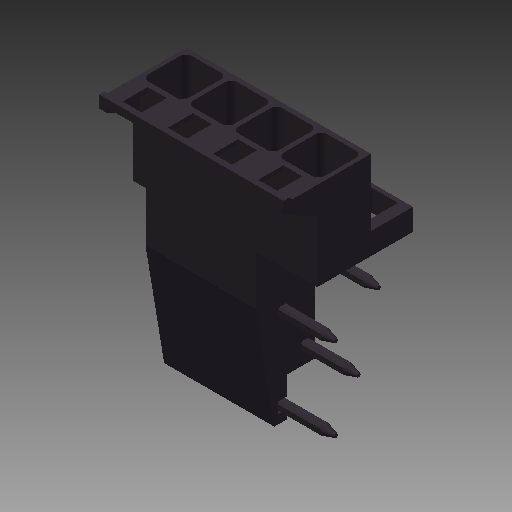
# Autodesk Inventor part: SHL-SMT5.00/04/GL 5.9BX 1069770000
Saved by Autodesk Inventor 2019.3 (Build 233278000, 278)
## iProperties
Category: PARTsolutions
Company: WEIDMUELLER
Created: 2018-11-15
Part Number: SHL-SMT5.00/04/GL 5.9BX 1069770000
Material: Generic
Catalog Web Link: www.cadenas.de
Description: SHL-SMT5.00/GL-Electronics housings
Vendor: WEIDMUELLER
Document SubType Name: Modeling
Designer: psadmin
Manufacturer: WEIDMUELLER
Mass: 1.86348 g
Surface Area: 26.7097 cm^2
Volume: 1.86348 cm^3
Density: 1 g/cm^3
Appearance: PSOLRGB-68-61-68
PSOL_IDENT_0: {$CADENAS_DATA\23d-libs\weidmueller\elektronikgehaeuse\einbaugehaeuse\ch20m\zubehoer\shl-smt500_gl.p
PSOL_IDENT_1: rj},216 {VTYP=3D},{NB=SHL-SMT5.00/04/GL 5.9BX 1069770000},{LINA=SHL-SMT5.00/04/GL 5.9BX 1069770000},
PSOL_IDENT_2: {NN=SHL-SMT5.00/GL},{DATE=31.03.2017 09:22:38},{GEOMDATE=25.06.2010 07:04:00},{VERSION=},{LINEID=50}
PSOL_IDENT_3: ,{WBVAR=},{WBNUMERIC=}  {NB=SHL-SMT5.00/04/GL 5.9BX 1069770000},{LINA=SHL-SMT5.00/04/GL 5.9BX 106977
PSOL_IDENT_4: 0000},{KT=DUMMY},{BEST=1069770000},{BZ=SHL-SMT5.00/04/GL 5.9BX},{R=5.00},{P=4},{L=5.90},{F=schwarz},
PSOL_IDENT_5: {FCODE=0.27,0.24,0.27,0.00}
NN: SHL-SMT5.00/GL
NT: Electronics housings
NB: SHL-SMT5.00/04/GL 5.9BX 1069770000
NBSYN: $BZ. $BEST.
LINA: SHL-SMT5.00/04/GL 5.9BX 1069770000
BEST: 1069770000
BZ: SHL-SMT5.00/04/GL 5.9BX
R: 5
P: 4
L: 5.9
F: black
SUPPLIER: WEIDMUELLER
ARTICLENO: SHL-SMT5.00/04/GL 5.9BX 1069770000
BOMINFO: SHL-SMT5.00/04/GL 5.9BX 1069770000
CREATOR: CADENAS GmbH
Title: SHL-SMT5.00/04/GL 5.9BX 1069770000
Author: Cadenas PARTsolutions
Comments: Electronics housings
Autodesk Inventor part; units mm, degrees
sketch "Sketch_2" plane through (-15.2, 0, 0) normal (1, 0, 0) x (0, 0, -1)
  line L0 (-14.35, 12.05) -> (-14.35, 10.7061)
  line L1 (-14.35, 10.7061) -> (-10.6, 8.67)
  line L2 (-10.6, 8.67) -> (-10.6, -3.6)
  line L3 (-10.6, -3.6) -> (-8.5417, -15.9)
  line L4 (-8.5417, -15.9) -> (-7.1, -15.9)
  line L5 (-7.1, -15.9) -> (-7.1, -11.6)
  line L6 (-7.1, -11.6) -> (-4.1, -11.6)
  line L7 (-4.1, -11.6) -> (-4.1, -4.05)
  line L8 (-4.1, -4.05) -> (-1.85, -4.05)
  line L9 (-1.85, -4.05) -> (-1.85, 1.9)
  line L10 (-1.85, 1.9) -> (0, 1.9)
  line L11 (0, 1.9) -> (0, 4.3)
  line L12 (0, 4.3) -> (-4.64, 4.3)
  line L13 (-4.64, 4.3) -> (-4.64, 11.7)
  line L14 (-4.64, 11.7) -> (-13.375, 11.7)
  line L15 (-13.375, 11.7) -> (-13.725, 12.05)
  line L16 (-13.725, 12.05) -> (-14.35, 12.05)
  constraints: 34 end point
extrude "Extrusion1" add sketch "Sketch_2" along normal blind 20.4
sketch "Sketch_4" plane through (0, 0, 0) normal (0, 0, 1) x (1, 0, 0)
  line L0 (-1.6, -16) -> (5.4, -16)
  line L1 (5.4, -16) -> (5.4, 1.9)
  line L2 (5.4, 1.9) -> (-1.6, 1.9)
  line L3 (-1.6, 1.9) -> (-1.6, -16)
  constraints: 8 end point
extrude "Extrusion2" cut sketch "Sketch_4" along normal blind 11
sketch "Sketch_15" plane through (0, 0, 0) normal (0, 0, 1) x (1, 0, 0)
  line L0 (-15.5, -5.1) -> (-6.5, -5.1)
  line L1 (-6.5, -5.1) -> (-6.5, 1.9)
  line L2 (-6.5, 1.9) -> (-15.5, 1.9)
  line L3 (-15.5, 1.9) -> (-15.5, -5.1)
  constraints: 8 end point
extrude "Extrusion3" cut sketch "Sketch_15" along normal blind 4.1
sketch "Sketch_13" plane through (0, 11.7, 0) normal (0, 1, 0) x (1, 0, 0)
  line L0 (0.25, -5.825) -> (0.25, -9.375)
  arc A0 (0.25, -9.375) -> (0.9, -10.025) centre (0.9, -9.375) ccw
  line L1 (0.9, -10.025) -> (4.1, -10.025)
  arc A1 (4.1, -10.025) -> (4.75, -9.375) centre (4.1, -9.375) ccw
  line L2 (4.75, -9.375) -> (4.75, -5.825)
  arc A2 (4.75, -5.825) -> (4.1, -5.175) centre (4.1, -5.825) ccw
  line L3 (4.1, -5.175) -> (0.9, -5.175)
  arc A3 (0.9, -5.175) -> (0.25, -5.825) centre (0.9, -5.825) ccw
  constraints: 8 end point, 8 point on circle, 4 centre point
extrude "Extrusion4" cut sketch "Sketch_13" against normal blind 8.7
pattern_linear "Rectangular Pattern1" count 4 spacing 5 along (-1, 0, 0) of "Extrusion4"
sketch "Sketch_21" plane through (0, 11.7, 0) normal (0, 1, 0) x (1, 0, 0)
  line L0 (1.45, -10.6) -> (1.45, -13.375)
  line L1 (1.45, -13.375) -> (3.55, -13.375)
  line L2 (3.55, -13.375) -> (3.55, -10.6)
  line L3 (3.55, -10.6) -> (1.45, -10.6)
  constraints: 8 end point
extrude "Extrusion5" cut sketch "Sketch_21" against normal blind 4
pattern_linear "Rectangular Pattern2" count 4 spacing 5 along (-1, 0, 0) of "Extrusion5"
sketch "Sketch_23" plane through (-14.4, 0, 0) normal (1, 0, 0) x (0, 0, -1)
  line L0 (-14.6, 8.2) -> (-10.6, 8.2)
  line L1 (-10.6, 8.2) -> (-10.6, 11.2)
  line L2 (-10.6, 11.2) -> (-14.6, 11.2)
  line L3 (-14.6, 11.2) -> (-14.6, 8.2)
  constraints: 8 end point
extrude "Extrusion6" cut sketch "Sketch_23" along normal blind 18.8
sketch "Sketch_28" plane through (0, 4.3, 0) normal (0, 1, 0) x (1, 0, 0)
  line L0 (1, -0.65) -> (1, -3.65)
  arc A0 (1, -3.65) -> (1.2, -3.85) centre (1.2, -3.65) ccw
  line L1 (1.2, -3.85) -> (3.8, -3.85)
  arc A1 (3.8, -3.85) -> (4, -3.65) centre (3.8, -3.65) ccw
  line L2 (4, -3.65) -> (4, -0.65)
  arc A2 (4, -0.65) -> (3.8, -0.45) centre (3.8, -0.65) ccw
  line L3 (3.8, -0.45) -> (1.2, -0.45)
  arc A3 (1.2, -0.45) -> (1, -0.65) centre (1.2, -0.65) ccw
  constraints: 8 end point, 8 point on circle, 4 centre point
extrude "Extrusion7" cut sketch "Sketch_28" against normal blind 2.4
sketch "Sketch_29" plane through (0, 4.3, 0) normal (0, 1, 0) x (1, 0, 0)
  line L0 (-14, -0.65) -> (-14, -3.65)
  arc A0 (-14, -3.65) -> (-13.8, -3.85) centre (-13.8, -3.65) ccw
  line L1 (-13.8, -3.85) -> (-11.2, -3.85)
  arc A1 (-11.2, -3.85) -> (-11, -3.65) centre (-11.2, -3.65) ccw
  line L2 (-11, -3.65) -> (-11, -0.65)
  arc A2 (-11, -0.65) -> (-11.2, -0.45) centre (-11.2, -0.65) ccw
  line L3 (-11.2, -0.45) -> (-13.8, -0.45)
  arc A3 (-13.8, -0.45) -> (-14, -0.65) centre (-13.8, -0.65) ccw
  constraints: 8 end point, 8 point on circle, 4 centre point
extrude "Extrusion8" cut sketch "Sketch_29" against normal blind 2.4
sketch "Sketch_10" plane through (0, 0, 7.1) normal (0, 0, 1) x (1, 0, 0)
  line L0 (-13.1, 1.9) -> (-13.1, -13.2)
  arc A0 (-13.1, -13.2) -> (-11.4, -14.9) centre (-11.4, -13.2) ccw
  line L1 (-11.4, -14.9) -> (-1.6, -14.9)
  line L2 (-1.6, -14.9) -> (-1.6, -13.7)
  line L3 (-1.6, -13.7) -> (-11.4, -13.7)
  arc A1 (-11.9, -13.2) -> (-11.4, -13.7) centre (-11.4, -13.2) ccw
  line L4 (-11.9, -13.2) -> (-11.9, 1.9)
  line L5 (-11.9, 1.9) -> (-13.1, 1.9)
  constraints: 12 end point, 4 point on circle, 2 centre point
extrude "Extrusion9" cut sketch "Sketch_10" along normal blind 1
sketch "Sketch_5" plane through (4.3, 0, 0) normal (1, 0, 0) x (0, 0, -1)
  line L0 (-8.1, -4.9) -> (-8.1, -5.5)
  line L1 (-8.1, -5.5) -> (-7.9, -5.7)
  line L2 (-7.9, -5.7) -> (-7.3, -5.7)
  line L3 (-7.3, -5.7) -> (-7.1, -5.5)
  line L4 (-7.1, -5.5) -> (-7.1, -4.9)
  line L5 (-7.1, -4.9) -> (-7.3, -4.7)
  line L6 (-7.3, -4.7) -> (-7.9, -4.7)
  line L7 (-7.9, -4.7) -> (-8.1, -4.9)
  constraints: 16 end point
extrude "Extrusion10" add sketch "Sketch_5" against normal blind 6.9
sketch "Sketch_6" plane through (4.3, 0, 0) normal (1, 0, 0) x (0, 0, -1)
  line L0 (-8.1, -14) -> (-8.1, -14.6)
  line L1 (-8.1, -14.6) -> (-7.9, -14.8)
  line L2 (-7.9, -14.8) -> (-7.3, -14.8)
  line L3 (-7.3, -14.8) -> (-7.1, -14.6)
  line L4 (-7.1, -14.6) -> (-7.1, -14)
  line L5 (-7.1, -14) -> (-7.3, -13.8)
  line L6 (-7.3, -13.8) -> (-7.9, -13.8)
  line L7 (-7.9, -13.8) -> (-8.1, -14)
  constraints: 16 end point
extrude "Extrusion11" add sketch "Sketch_6" against normal blind 15.7
sketch "Sketch_11" plane through (-11.4, 0, 0) normal (1, 0, 0) x (0, 0, -1)
  line L0 (-7.9, -13.2) -> (-7.3, -13.2)
  line L1 (-8.1, -14) -> (-8.1, -14.6)
  line L2 (-8.1, -14.6) -> (-7.9, -14.8)
  line L3 (-7.9, -14.8) -> (-7.3, -14.8)
  line L4 (-7.3, -14.8) -> (-7.1, -14.6)
  line L5 (-7.1, -14.6) -> (-7.1, -14)
  line L6 (-7.1, -14) -> (-7.3, -13.8)
  line L7 (-7.3, -13.8) -> (-7.9, -13.8)
  line L8 (-7.9, -13.8) -> (-8.1, -14)
  constraints: 18 end point
revolve "Revolution1" add sketch "Sketch_11" angle 90 about axis through (-11.4, -13.2, 7.9) along (0, 0, -1)
sketch "Sketch_12" plane through (0, -13.2, 0) normal (0, 1, 0) x (1, 0, 0)
  line L0 (-13, -7.9) -> (-12.8, -8.1)
  line L1 (-12.8, -8.1) -> (-12.2, -8.1)
  line L2 (-12.2, -8.1) -> (-12, -7.9)
  line L3 (-12, -7.9) -> (-12, -7.3)
  line L4 (-12, -7.3) -> (-12.2, -7.1)
  line L5 (-12.2, -7.1) -> (-12.8, -7.1)
  line L6 (-12.8, -7.1) -> (-13, -7.3)
  line L7 (-13, -7.3) -> (-13, -7.9)
  constraints: 16 end point
extrude "Extrusion12" add sketch "Sketch_12" along normal blind 22.7
sketch "Sketch_7" plane through (4.3, 0, 0) normal (1, 0, 0) x (0, 0, -1)
  line L0 (-3.35, -2.2) -> (-3.35, -2.8)
  line L1 (-3.35, -2.8) -> (-3.15, -3)
  line L2 (-3.15, -3) -> (-2.55, -3)
  line L3 (-2.55, -3) -> (-2.35, -2.8)
  line L4 (-2.35, -2.8) -> (-2.35, -2.2)
  line L5 (-2.35, -2.2) -> (-2.55, -2)
  line L6 (-2.55, -2) -> (-3.15, -2)
  line L7 (-3.15, -2) -> (-3.35, -2.2)
  constraints: 16 end point
extrude "Extrusion13" add sketch "Sketch_7" against normal blind 6.9
sketch "Sketch_8" plane through (4.3, 0, 0) normal (1, 0, 0) x (0, 0, -1)
  line L0 (-5.6, -9.45) -> (-5.6, -10.05)
  line L1 (-5.6, -10.05) -> (-5.4, -10.25)
  line L2 (-5.4, -10.25) -> (-4.8, -10.25)
  line L3 (-4.8, -10.25) -> (-4.6, -10.05)
  line L4 (-4.6, -10.05) -> (-4.6, -9.45)
  line L5 (-4.6, -9.45) -> (-4.8, -9.25)
  line L6 (-4.8, -9.25) -> (-5.4, -9.25)
  line L7 (-5.4, -9.25) -> (-5.6, -9.45)
  constraints: 16 end point
extrude "Extrusion14" add sketch "Sketch_8" against normal blind 6.9
sketch "Sketch_17" plane through (0, 9.5, 0) normal (0, 1, 0) x (1, 0, 0)
  line L0 (-8, -7.9) -> (-7.8, -8.1)
  line L1 (-7.8, -8.1) -> (-7.2, -8.1)
  line L2 (-7.2, -8.1) -> (-7, -7.9)
  line L3 (-7, -7.9) -> (-7, -7.3)
  line L4 (-7, -7.3) -> (-7.2, -7.1)
  line L5 (-7.2, -7.1) -> (-7.8, -7.1)
  line L6 (-7.8, -7.1) -> (-8, -7.3)
  line L7 (-8, -7.3) -> (-8, -7.9)
  constraints: 16 end point
extrude "Extrusion15" add sketch "Sketch_17" against normal blind 7
sketch "Sketch_16" plane through (0, 9.5, 0) normal (0, 1, 0) x (1, 0, 0)
  line L0 (-3, -7.9) -> (-2.8, -8.1)
  line L1 (-2.8, -8.1) -> (-2.2, -8.1)
  line L2 (-2.2, -8.1) -> (-2, -7.9)
  line L3 (-2, -7.9) -> (-2, -7.3)
  line L4 (-2, -7.3) -> (-2.2, -7.1)
  line L5 (-2.2, -7.1) -> (-2.8, -7.1)
  line L6 (-2.8, -7.1) -> (-3, -7.3)
  line L7 (-3, -7.3) -> (-3, -7.9)
  constraints: 16 end point
extrude "Extrusion16" add sketch "Sketch_16" against normal blind 7
sketch "Sketch_18" plane through (0, 9.5, 0) normal (0, 1, 0) x (1, 0, 0)
  line L0 (2, -7.9) -> (2.2, -8.1)
  line L1 (2.2, -8.1) -> (2.8, -8.1)
  line L2 (2.8, -8.1) -> (3, -7.9)
  line L3 (3, -7.9) -> (3, -7.3)
  line L4 (3, -7.3) -> (2.8, -7.1)
  line L5 (2.8, -7.1) -> (2.2, -7.1)
  line L6 (2.2, -7.1) -> (2, -7.3)
  line L7 (2, -7.3) -> (2, -7.9)
  constraints: 16 end point
extrude "Extrusion17" add sketch "Sketch_18" against normal blind 7
sketch "Sketch_19" plane through (0, 0, 7.6) normal (0, 0, 1) x (1, 0, 0)
  line L0 (2.5, 8.1) -> (2.5, 9.7931)
  line L1 (2.5, 9.7) -> (3.3, 9.7)
  line L2 (3.3, 9.7) -> (3.3, 8.1)
  line L3 (3.3, 8.1) -> (3.1, 8.1)
  line L4 (3.1, 8.1) -> (2.7, 9.5)
  line L5 (2.7, 9.5) -> (2.5, 9.5)
  line L6 (2.5, 9.5) -> (2.5, 9.7)
  constraints: 14 end point
revolve "Revolution2" cut sketch "Sketch_19" angle 360 about axis through (2.5, 8.1, 7.6) along (0, -1, 0)
pattern_linear "Rectangular Pattern3" count 4 spacing 5 along (-1, 0, 0) of "Revolution2"
sketch "Sketch_24" plane through (0, 0, 7.6) normal (0, 0, 1) x (1, 0, 0)
  line L0 (2.9, -5.2) -> (4.5931, -5.2)
  line L1 (4.5, -5.2) -> (4.5, -6)
  line L2 (4.5, -6) -> (2.9, -6)
  line L3 (2.9, -6) -> (2.9, -5.8)
  line L4 (2.9, -5.8) -> (4.3, -5.4)
  line L5 (4.3, -5.4) -> (4.3, -5.2)
  line L6 (4.3, -5.2) -> (4.5, -5.2)
  constraints: 14 end point
revolve "Revolution3" cut sketch "Sketch_24" angle 360 about axis through (2.9, -5.2, 7.6) along (-1, 0, 0)
sketch "Sketch_25" plane through (0, 0, 7.6) normal (0, 0, 1) x (1, 0, 0)
  line L0 (2.9, -14.3) -> (4.5931, -14.3)
  line L1 (4.5, -14.3) -> (4.5, -15.1)
  line L2 (4.5, -15.1) -> (2.9, -15.1)
  line L3 (2.9, -15.1) -> (2.9, -14.9)
  line L4 (2.9, -14.9) -> (4.3, -14.5)
  line L5 (4.3, -14.5) -> (4.3, -14.3)
  line L6 (4.3, -14.3) -> (4.5, -14.3)
  constraints: 14 end point
revolve "Revolution4" cut sketch "Sketch_25" angle 360 about axis through (2.9, -14.3, 7.6) along (-1, 0, 0)
sketch "Sketch_26" plane through (0, 0, 5.1) normal (0, 0, 1) x (1, 0, 0)
  line L0 (2.9, -9.75) -> (4.5931, -9.75)
  line L1 (4.5, -9.75) -> (4.5, -10.55)
  line L2 (4.5, -10.55) -> (2.9, -10.55)
  line L3 (2.9, -10.55) -> (2.9, -10.35)
  line L4 (2.9, -10.35) -> (4.3, -9.95)
  line L5 (4.3, -9.95) -> (4.3, -9.75)
  line L6 (4.3, -9.75) -> (4.5, -9.75)
  constraints: 14 end point
revolve "Revolution5" cut sketch "Sketch_26" angle 360 about axis through (2.9, -9.75, 5.1) along (-1, 0, 0)
sketch "Sketch_27" plane through (0, 0, 2.85) normal (0, 0, 1) x (1, 0, 0)
  line L0 (2.9, -2.5) -> (4.5931, -2.5)
  line L1 (4.5, -2.5) -> (4.5, -3.3)
  line L2 (4.5, -3.3) -> (2.9, -3.3)
  line L3 (2.9, -3.3) -> (2.9, -3.1)
  line L4 (2.9, -3.1) -> (4.3, -2.7)
  line L5 (4.3, -2.7) -> (4.3, -2.5)
  line L6 (4.3, -2.5) -> (4.5, -2.5)
  constraints: 14 end point
revolve "Revolution6" cut sketch "Sketch_27" angle 360 about axis through (2.9, -2.5, 2.85) along (-1, 0, 0)
sketch "Sketch_31" plane through (0, 0, 0) normal (0, 0, 1) x (1, 0, 0)
  line L0 (-15.2, 1.9) -> (-15.2, -16.1)
  line L1 (-15.2, -16.1) -> (-13.8, -16.1)
  line L2 (-13.8, -16.1) -> (-13.8, 1.9)
  line L3 (-13.8, 1.9) -> (-15.2, 1.9)
  constraints: 8 end point
extrude "Extrusion18" cut sketch "Sketch_31" along normal blind 12
ref_plane "mitBHZ_XY" through (2.5, 11.7, 7.6) normal (0, -1, 0) x (1, 0, 0)
ref_plane "mitBHZ_YZ" through (2.5, 11.7, 7.6) normal (1, 0, 0) x (0, 0, 1)
ref_plane "mitBHZ_ZX" through (2.5, 11.7, 7.6) normal (0, 0, 1) x (0, -1, 0)
ref_plane "mitPCB_XY" through (0, -2.5, 2.85) normal (1, 0, 0) x (0, 0, -1)
ref_plane "mitPCB_YZ" through (0, -2.5, 2.85) normal (0, 0, -1) x (0, 1, 0)
ref_plane "mitPCB_ZX" through (0, -2.5, 2.85) normal (0, 1, 0) x (1, 0, 0)
body "Solid1"
